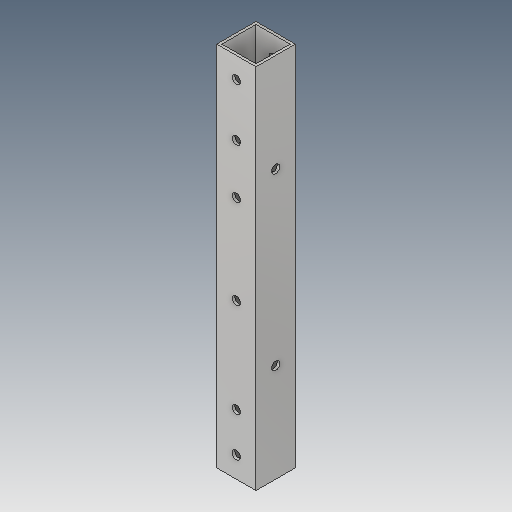
# Autodesk Inventor part: PitchSquarePipe2
Saved by Autodesk Inventor 2019.4 (Build 234330000, 330)
## iProperties
Created: 2019-06-11
Part Number: PitchSquarePipe2
Material: アルミニウム 5005-H12
Document SubType Name: Modeling
Designer: AzLIer
Density: 2.7 g/cm^3
Appearance: アルミニウム - つや出し
Mass: 20.9943 g
Surface Area: 157.437 cm^2
Volume: 7.77566 cm^3
Author: AzLIer
Autodesk Inventor part; units mm, degrees
ref_plane "YZ Plane" through (0, 0, 0) normal (1, 0, 0) x (0, 1, 0)
ref_plane "XZ Plane" through (0, 0, 0) normal (0, 1, 0) x (-1, 0, 0)
ref_plane "XY Plane" through (0, 0, 0) normal (0, 0, 1) x (1, 0, 0)
sketch "スケッチ1" plane through (0, 0, 0) normal (0, 1, 0) x (-1, 0, 0)
  line L0 (7.5, -7.5) -> (-7.5, -7.5)
  line L1 (-7.5, -7.5) -> (-7.5, 7.5)
  line L2 (-7.5, 7.5) -> (7.5, 7.5)
  line L3 (7.5, 7.5) -> (7.5, -7.5)
  line L4 (7.5, -7.5) -> (-7.5, 7.5) construction
  line L5 (-7.5, -7.5) -> (7.5, 7.5) construction
  point P0 (0, 0)
  dimension "d0" = 15
  dimension "d1" = 15
  constraints: 12 end point, 2 midpoint, 2 parallel, 1 horizontal, 1 perpendicular
  measures "d0" distance of L1.end L2.end
  measures "d1" distance of L0.end L1.end
extrude "押し出し1" add sketch "スケッチ1" along normal blind 140
shell "シェル1" thickness 1 removed faces 2 at (-2.5, 0, -2.5) at (-2.5, 140, -2.5)
sketch "スケッチ2" plane through (-7.5, 0, 7.5) normal (0, 0, 1) x (1, 0, 0)
  line L0 (15, 0) -> (0, 0) projected
  line L1 (0, 140) -> (15, 140) projected
  point P0 (7.5, 0)
  point P1 (7.5, 8)
  point P2 (7.5, 23)
  point P3 (7.5, 0)
  point P4 (7.5, 132)
  point P5 (7.5, 112)
  point P6 (7.5, 140)
  dimension "d5" = 8
  dimension "d6" = 15
  dimension "d14" = 8
  dimension "d15" = 20
  constraints: 4 vertical alignment, 2 midpoint
  measures "d5" distance of point (7.5, 0) point (7.5, 8)
  measures "d6" distance of point (7.5, 23) point (7.5, 8)
  measures "d14" distance from line of L1 point (7.5, 132)
  measures "d15" distance of point (7.5, 112) point (7.5, 132)
hole "穴1" at (0, 8, 7.5) at (0, 23, 7.5) at (0, 132, 7.5) at (0, 112, 7.5) direction (0, 0, -1) diameter 3.2 end through all
sketch "スケッチ3" plane through (-7.5, 0, -7.5) normal (-1, 0, 0) x (0, 0, 1)
  line L0 (15, 0) -> (0, 0) projected
  point P0 (7.5, 0)
  point P1 (7.5, 37.5)
  point P2 (7.5, 102.5)
  point P3 (7.5, 0)
  point P4 (7.5, 0)
  dimension "d16" = 37.5
  dimension "d17" = 65
  constraints: 2 midpoint, 2 vertical alignment
  measures "d16" distance from line of L0 point (7.5, 37.5)
  measures "d17" distance of point (7.5, 102.5) point (7.5, 37.5)
hole "穴2" at (-7.5, 37.5, 0) at (-7.5, 102.5, 0) direction (1, 0, 0) diameter 3.2 end through all
sketch "スケッチ4" plane through (-7.5, 0, 7.5) normal (0, 0, 1) x (1, 0, 0)
  circle A0 centre (94.8138, 137.4022) radius 1.6
  circle A1 centre (-2.6682, 183.8917) radius 1.6
  circle A2 centre (99.3065, 100.3608) radius 1.6
  circle A3 centre (1.8246, 146.8503) radius 1.6
  circle A4 centre (7.5, 112) radius 1.2295
  circle A5 centre (7.5, 132) radius 1.2295
  line L0 (112.2687, 136.8332) -> (109.5609, 138.1246)
  arc A6 (110.4218, 139.9298) -> (109.5609, 138.1246) centre (109.9914, 139.0272) ccw
  line L1 (110.4218, 139.9298) -> (112.1436, 143.5402)
  arc A7 (113.8704, 143.6762) -> (112.1436, 143.5402) centre (113.0463, 143.1098) ccw
  arc A8 (114.8515, 142.2489) -> (113.8704, 143.6762) centre (113.9489, 142.6793) ccw
  line L2 (114.8515, 142.2489) -> (113.1296, 138.6384)
  arc A9 (112.2687, 136.8332) -> (113.1296, 138.6384) centre (112.6992, 137.7358) ccw
  line L3 (120.017, 153.0802) -> (118.2951, 149.4697)
  arc A10 (116.5684, 149.3337) -> (118.2951, 149.4697) centre (117.3925, 149.9002) ccw
  arc A11 (115.5873, 150.7611) -> (116.5684, 149.3337) centre (116.4899, 150.3307) ccw
  line L4 (115.5873, 150.7611) -> (117.3091, 154.3716)
  arc A12 (118.1701, 156.1768) -> (117.3091, 154.3716) centre (117.7396, 155.2742) ccw
  line L5 (118.1701, 156.1768) -> (120.8779, 154.8854)
  arc A13 (120.017, 153.0802) -> (120.8779, 154.8854) centre (120.4474, 153.9828) ccw
  line L6 (106.2423, 124.1966) -> (103.5345, 125.488)
  arc A14 (104.3954, 127.2932) -> (103.5345, 125.488) centre (103.9649, 126.3906) ccw
  line L7 (104.3954, 127.2932) -> (106.1172, 130.9037)
  arc A15 (107.8439, 131.0397) -> (106.1172, 130.9037) centre (107.0198, 130.4732) ccw
  arc A16 (108.8251, 129.6123) -> (107.8439, 131.0397) centre (107.9225, 130.0428) ccw
  line L8 (108.8251, 129.6123) -> (107.1032, 126.0019)
  arc A17 (106.2423, 124.1966) -> (107.1032, 126.0019) centre (106.6728, 125.0992) ccw
  circle A18 centre (51.5477, 186.0658) radius 1.6
  circle A19 centre (60.463, 120.5473) radius 1.5
  circle A20 centre (40.987, 157.5329) radius 1.5
  circle A21 centre (30.2256, 134.9676) radius 1.5
  circle A22 centre (71.2245, 143.1126) radius 1.5
  circle A23 centre (72.3508, 176.2555) radius 1.25
  circle A24 centre (94.0134, 165.9245) radius 1.25
  arc A25 (80.796, 100.4622) -> (79.0196, 101.3811) centre (79.9078, 100.9217) ccw
  line L9 (80.796, 100.4622) -> (75.2827, 89.8038)
  arc A26 (73.5063, 90.7226) -> (75.2827, 89.8038) centre (74.3945, 90.2632) ccw
  line L10 (73.5063, 90.7226) -> (64.6242, 95.3171)
  arc A27 (62.8478, 96.2359) -> (64.6242, 95.3171) centre (63.736, 95.7765) ccw
  line L11 (62.8478, 96.2359) -> (68.3611, 106.8944)
  arc A28 (70.1375, 105.9755) -> (68.3611, 106.8944) centre (69.2493, 106.435) ccw
  line L12 (70.1375, 105.9755) -> (79.0196, 101.3811)
  circle A29 centre (28.7854, 103.2592) radius 1.5
  circle A30 centre (67.6869, 90.3552) radius 1.5
  circle A31 centre (75.9568, 106.343) radius 1.5
  circle A32 centre (31.7101, 121.02) radius 1.5
  line L13 (38.1296, 116.9224) -> (36.1798, 105.0819)
  arc A33 (34.2064, 105.4069) -> (36.1798, 105.0819) centre (35.1931, 105.2444) ccw
  line L14 (34.2064, 105.4069) -> (24.3393, 107.0317)
  arc A34 (22.3659, 107.3567) -> (24.3393, 107.0317) centre (23.3526, 107.1942) ccw
  line L15 (22.3659, 107.3567) -> (24.3157, 119.1972)
  arc A35 (26.2891, 118.8723) -> (24.3157, 119.1972) centre (25.3024, 119.0347) ccw
  line L16 (26.2891, 118.8723) -> (36.1562, 117.2474)
  arc A36 (38.1296, 116.9224) -> (36.1562, 117.2474) centre (37.1429, 117.0849) ccw
  circle A37 centre (-0.9114, 173.6368) radius 1.6
  circle A38 centre (91.1549, 129.73) radius 1.6
  arc A39 (89.211, 114.0386) -> (91.0163, 113.1777) centre (90.1137, 113.6081) ccw
  line L17 (89.211, 114.0386) -> (80.1849, 118.3432)
  arc A40 (78.3797, 119.2041) -> (80.1849, 118.3432) centre (79.2823, 118.7736) ccw
  line L18 (78.3797, 119.2041) -> (83.5452, 130.0354)
  arc A41 (85.3504, 129.1745) -> (83.5452, 130.0354) centre (84.4478, 129.605) ccw
  line L19 (85.3504, 129.1745) -> (94.3765, 124.8699)
  arc A42 (96.1818, 124.009) -> (94.3765, 124.8699) centre (95.2792, 124.4395) ccw
  line L20 (96.1818, 124.009) -> (91.0163, 113.1777)
  arc A43 (-6.7159, 173.0812) -> (-8.5211, 173.9421) centre (-7.6185, 173.5117) ccw
  line L21 (-6.7159, 173.0812) -> (2.3103, 168.7766)
  arc A44 (4.1155, 167.9157) -> (2.3103, 168.7766) centre (3.2129, 168.3462) ccw
  line L22 (4.1155, 167.9157) -> (-1.05, 157.0844)
  arc A45 (-2.8552, 157.9453) -> (-1.05, 157.0844) centre (-1.9526, 157.5148) ccw
  line L23 (-2.8552, 157.9453) -> (-11.8813, 162.2499)
  arc A46 (-13.6866, 163.1108) -> (-11.8813, 162.2499) centre (-12.784, 162.6803) ccw
  line L24 (-13.6866, 163.1108) -> (-8.5211, 173.9421)
  circle A47 centre (83.4066, 113.4831) radius 1.6
  circle A48 centre (-8.6597, 157.3898) radius 1.6
  circle A49 centre (9.0871, 193.022) radius 1.25
  circle A50 centre (11.8045, 158.4877) radius 1.25
  circle A51 centre (40.3533, 178.1082) radius 1.25
  circle A52 centre (60.4103, 159.3488) radius 1.2295
  circle A53 centre (78.2541, 161.9181) radius 1.2295
  circle A54 centre (51.1757, 174.8318) radius 1.2295
  arc A55 (-2.9, 96) -> (-6, 96) centre (-4.45, 96) ccw
  line L25 (-2.9, 96) -> (-2.9, 90)
  arc A56 (-6, 90) -> (-2.9, 90) centre (-4.45, 90) ccw
  line L26 (-6, 90) -> (-6, 96)
  circle A57 centre (49.5584, 72.8565) radius 1.6
  circle A58 centre (7.5, 59) radius 1.25
  circle A59 centre (7.5, 93) radius 1.25
  arc A60 (-2.9, 62) -> (-6, 62) centre (-4.45, 62) ccw
  line L27 (-2.9, 62) -> (-2.9, 56)
  arc A61 (-6, 56) -> (-2.9, 56) centre (-4.45, 56) ccw
  line L28 (-6, 56) -> (-6, 62)
  arc A62 (0, 103) -> (0, 106) centre (0, 104.5) ccw
  line L29 (-9, 103) -> (0, 103)
  line L30 (-9, 83) -> (-9, 103)
  line L31 (0, 83) -> (-9, 83)
  arc A63 (0, 80) -> (0, 83) centre (0, 81.5) ccw
  line L32 (0, 80) -> (0, 72)
  arc A64 (0, 69) -> (0, 72) centre (0, 70.5) ccw
  line L33 (-9, 69) -> (0, 69)
  line L34 (-9, 49) -> (-9, 69)
  line L35 (0, 49) -> (-9, 49)
  arc A65 (0, 46) -> (0, 49) centre (0, 47.5) ccw
  line L36 (0, 46) -> (0, 42)
  arc A66 (0, 42) -> (1.4237, 42.3594) centre (0, 45) ccw
  line L37 (1.4237, 42.3594) -> (101.4896, 96.3119)
  arc A67 (101.4896, 96.3119) -> (103.6033, 98.7183) centre (99.3065, 100.3608) ccw
  line L38 (124.1837, 152.5545) -> (103.6033, 98.7183)
  arc A68 (124.1837, 152.5545) -> (122.1359, 157.6089) centre (120.4474, 153.9828) ccw
  line L39 (53.2362, 189.6919) -> (122.1359, 157.6089)
  arc A69 (53.2362, 189.6919) -> (48.9495, 189.107) centre (51.5477, 186.0658) ccw
  line L40 (38.5483, 180.221) -> (48.9495, 189.107)
  arc A70 (38.5483, 180.221) -> (37.5746, 178.1426) centre (40.3533, 178.1082) ccw
  arc A71 (35.9884, 171.3281) -> (37.5746, 178.1426) centre (21.2759, 178.3445) ccw
  line L41 (35.9884, 171.3281) -> (35.1275, 169.5229)
  arc A72 (5.7024, 183.5558) -> (35.1275, 169.5229) centre (20.415, 176.5393) ccw
  line L42 (5.7024, 183.5558) -> (6.5633, 185.361)
  arc A73 (10.8623, 190.8844) -> (6.5633, 185.361) centre (21.2759, 178.3445) ccw
  arc A74 (10.8623, 190.8844) -> (7.898, 195.5334) centre (9.0871, 193.022) ccw
  line L43 (-5.2359, 189.3145) -> (7.898, 195.5334)
  arc A75 (-5.2359, 189.3145) -> (-8.284, 186.0042) centre (-2.6682, 183.8917) ccw
  line L44 (-16.5278, 164.0887) -> (-8.284, 186.0042)
  arc A76 (-16.5278, 164.0887) -> (-16.5876, 161.4424) centre (-12.784, 162.6803) ccw
  line L45 (-16.5876, 161.4424) -> (-0.1473, 110.9284)
  arc A77 (0, 110) -> (-0.1473, 110.9284) centre (-3, 110) ccw
  line L46 (0, 110) -> (0, 106)
  point P0 (7.5, 0)
  constraints: 96 point on circle, 94 end point, 78 centre point
hole "穴3" at (0, 59, 7.5) at (0, 93, 7.5) direction (0, 0, -1) diameter 3.2 end through all
